Autodesk Fusion 360 part; units mm, degrees
(part 2 of 3)
  spline S17 degree 5 poles (8.5092, -53.844) (8.509, -53.837) (8.5085, -53.8231) (8.5078, -53.8022) (8.5068, -53.7744) (8.5054, -53.7397) (8.5038, -53.7051) (8.5021, -53.6705) (8.5002, -53.6359) (8.4982, -53.6014) (8.496, -53.567) (8.4936, -53.5327) (8.4911, -53.4983) (8.4885, -53.4641) (8.4857, -53.4299) (8.4827, -53.3958) (8.4796, -53.3617) (8.4763, -53.3277) (8.4729, -53.2938) (8.4693, -53.2599) (8.4656, -53.2261) (8.4617, -53.1924) (8.4576, -53.1587) (8.4534, -53.1251) (8.449, -53.0916) (8.4444, -53.0581) (8.4397, -53.0248) (8.4348, -52.9914) (8.4298, -52.9582) (8.4245, -52.925) (8.4191, -52.892) (8.4136, -52.859) (8.4078, -52.826) (8.4019, -52.7932) (8.3958, -52.7604) (8.3896, -52.7278) (8.3832, -52.6952) (8.3765, -52.6627) (8.3697, -52.6302) (8.3628, -52.5979) (8.3556, -52.5657) (8.3483, -52.5335) (8.3407, -52.5015) (8.333, -52.4695) (8.3251, -52.4377) (8.3169, -52.4059) (8.3086, -52.3743) (8.3001, -52.3428) (8.2914, -52.3113) (8.2825, -52.28) (8.2734, -52.2488) (8.2641, -52.2177) (8.2545, -52.1867) (8.2447, -52.1559) (8.2346, -52.1252) (8.2244, -52.0946) (8.2139, -52.0641) (8.2032, -52.0338) (8.1924, -52.0035) (8.1812, -51.9735) (8.1698, -51.9436) (8.158, -51.9139) (8.1459, -51.8844) (8.1334, -51.8551) (8.1205, -51.826) (8.1075, -51.7971) (8.0943, -51.7683) (8.0808, -51.7396) (8.0672, -51.7111) (8.0531, -51.6829) (8.0382, -51.6551) (8.0255, -51.6334) (8.0154, -51.6175) (8.0083, -51.6071) (8.0048, -51.6019) knots -1 -1 -1 -1 -1 -1 -0.98571429 -0.97142857 -0.95714286 -0.94285714 -0.92857143 -0.91428571 -0.9 -0.88571429 -0.87142857 -0.85714286 -0.84285714 -0.82857143 -0.81428571 -0.8 -0.78571429 -0.77142857 -0.75714286 -0.74285714 -0.72857143 -0.71428571 -0.7 -0.68571429 -0.67142857 -0.65714286 -0.64285714 -0.62857143 -0.61428571 -0.6 -0.58571429 -0.57142857 -0.55714286 -0.54285714 -0.52857143 -0.51428571 -0.5 -0.48571429 -0.47142857 -0.45714286 -0.44285714 -0.42857143 -0.41428571 -0.4 -0.38571429 -0.37142857 -0.35714286 -0.34285714 -0.32857143 -0.31428571 -0.3 -0.28571429 -0.27142857 -0.25714286 -0.24285714 -0.22857143 -0.21428571 -0.2 -0.18571429 -0.17142857 -0.15714286 -0.14285714 -0.12857143 -0.11428571 -0.1 -0.08571429 -0.07142857 -0.05714286 -0.04285714 -0.02857143 -0.01428571 0 0 0 0 0 0
  line L17 (8.0048, -51.6019) -> (7.7787, -51.2734)
  arc A35 (7.8389, -50.9285) -> (7.7787, -51.2734) centre (7.9847, -51.1316) ccw
  arc A36 (7.8389, -50.9285) -> (8.5272, -50.4003) centre (0, -40) ccw
  arc A37 (8.876, -50.4314) -> (8.5272, -50.4003) centre (8.6858, -50.5937) ccw
  line L18 (8.876, -50.4314) -> (9.1348, -50.7348)
  spline S18 degree 5 poles (9.1348, -50.7348) (9.1388, -50.7396) (9.1471, -50.7491) (9.1599, -50.7629) (9.1775, -50.7809) (9.2005, -50.8024) (9.2241, -50.8234) (9.2481, -50.8439) (9.2724, -50.8643) (9.2968, -50.8845) (9.3213, -50.9046) (9.3461, -50.9245) (9.3711, -50.9442) (9.3965, -50.9636) (9.4221, -50.9826) (9.448, -51.0014) (9.4742, -51.02) (9.5006, -51.0383) (9.5271, -51.0565) (9.5539, -51.0744) (9.5807, -51.0923) (9.6078, -51.1099) (9.635, -51.1274) (9.6625, -51.1446) (9.6901, -51.1617) (9.7179, -51.1786) (9.7458, -51.1953) (9.7739, -51.2119) (9.8022, -51.2282) (9.8306, -51.2444) (9.8592, -51.2605) (9.8879, -51.2764) (9.9168, -51.2921) (9.9458, -51.3077) (9.9749, -51.3231) (10.0042, -51.3384) (10.0336, -51.3535) (10.0632, -51.3685) (10.0929, -51.3833) (10.1227, -51.3979) (10.1526, -51.4124) (10.1827, -51.4268) (10.2129, -51.441) (10.2432, -51.455) (10.2736, -51.4689) (10.3042, -51.4827) (10.3349, -51.4963) (10.3657, -51.5098) (10.3966, -51.5232) (10.4276, -51.5364) (10.4588, -51.5494) (10.49, -51.5624) (10.5214, -51.5751) (10.5528, -51.5878) (10.5844, -51.6003) (10.6161, -51.6127) (10.6479, -51.6249) (10.6798, -51.637) (10.7118, -51.6489) (10.7438, -51.6608) (10.776, -51.6725) (10.8083, -51.684) (10.8407, -51.6954) (10.8732, -51.7067) (10.9058, -51.7179) (10.9385, -51.7289) (10.9713, -51.7398) (11.0042, -51.7505) (11.0371, -51.7612) (11.0702, -51.7717) (11.1033, -51.782) (11.1299, -51.7902) (11.1499, -51.7963) (11.1633, -51.8003) (11.1699, -51.8023) knots 0 0 0 0 0 0 0.01428571 0.02857143 0.04285714 0.05714286 0.07142857 0.08571429 0.1 0.11428571 0.12857143 0.14285714 0.15714286 0.17142857 0.18571429 0.2 0.21428571 0.22857143 0.24285714 0.25714286 0.27142857 0.28571429 0.3 0.31428571 0.32857143 0.34285714 0.35714286 0.37142857 0.38571429 0.4 0.41428571 0.42857143 0.44285714 0.45714286 0.47142857 0.48571429 0.5 0.51428571 0.52857143 0.54285714 0.55714286 0.57142857 0.58571429 0.6 0.61428571 0.62857143 0.64285714 0.65714286 0.67142857 0.68571429 0.7 0.71428571 0.72857143 0.74285714 0.75714286 0.77142857 0.78571429 0.8 0.81428571 0.82857143 0.84285714 0.85714286 0.87142857 0.88571429 0.9 0.91428571 0.92857143 0.94285714 0.95714286 0.97142857 0.98571429 1 1 1 1 1 1
  arc A38 (11.1699, -51.8023) -> (11.8023, -51.1699) centre (0, -40) ccw
  spline S19 degree 5 poles (11.8023, -51.1699) (11.8003, -51.1633) (11.7963, -51.1499) (11.7902, -51.1299) (11.782, -51.1033) (11.7717, -51.0702) (11.7612, -51.0371) (11.7505, -51.0042) (11.7398, -50.9713) (11.7289, -50.9385) (11.7179, -50.9058) (11.7067, -50.8732) (11.6954, -50.8407) (11.684, -50.8083) (11.6725, -50.776) (11.6608, -50.7438) (11.6489, -50.7118) (11.637, -50.6798) (11.6249, -50.6479) (11.6127, -50.6161) (11.6003, -50.5844) (11.5878, -50.5528) (11.5751, -50.5214) (11.5624, -50.49) (11.5494, -50.4588) (11.5364, -50.4276) (11.5232, -50.3966) (11.5098, -50.3657) (11.4963, -50.3349) (11.4827, -50.3042) (11.4689, -50.2736) (11.455, -50.2432) (11.441, -50.2129) (11.4268, -50.1827) (11.4124, -50.1526) (11.3979, -50.1227) (11.3833, -50.0929) (11.3685, -50.0632) (11.3535, -50.0336) (11.3384, -50.0042) (11.3231, -49.9749) (11.3077, -49.9458) (11.2921, -49.9168) (11.2764, -49.8879) (11.2605, -49.8592) (11.2444, -49.8306) (11.2282, -49.8022) (11.2119, -49.7739) (11.1953, -49.7458) (11.1786, -49.7179) (11.1617, -49.6901) (11.1446, -49.6625) (11.1274, -49.635) (11.1099, -49.6078) (11.0923, -49.5807) (11.0744, -49.5539) (11.0565, -49.5271) (11.0383, -49.5006) (11.02, -49.4742) (11.0014, -49.448) (10.9826, -49.4221) (10.9636, -49.3965) (10.9442, -49.3711) (10.9245, -49.3461) (10.9046, -49.3213) (10.8845, -49.2968) (10.8643, -49.2724) (10.8439, -49.2481) (10.8234, -49.2241) (10.8024, -49.2005) (10.7809, -49.1775) (10.7629, -49.1599) (10.7491, -49.1471) (10.7396, -49.1388) (10.7348, -49.1348) knots -1 -1 -1 -1 -1 -1 -0.98571429 -0.97142857 -0.95714286 -0.94285714 -0.92857143 -0.91428571 -0.9 -0.88571429 -0.87142857 -0.85714286 -0.84285714 -0.82857143 -0.81428571 -0.8 -0.78571429 -0.77142857 -0.75714286 -0.74285714 -0.72857143 -0.71428571 -0.7 -0.68571429 -0.67142857 -0.65714286 -0.64285714 -0.62857143 -0.61428571 -0.6 -0.58571429 -0.57142857 -0.55714286 -0.54285714 -0.52857143 -0.51428571 -0.5 -0.48571429 -0.47142857 -0.45714286 -0.44285714 -0.42857143 -0.41428571 -0.4 -0.38571429 -0.37142857 -0.35714286 -0.34285714 -0.32857143 -0.31428571 -0.3 -0.28571429 -0.27142857 -0.25714286 -0.24285714 -0.22857143 -0.21428571 -0.2 -0.18571429 -0.17142857 -0.15714286 -0.14285714 -0.12857143 -0.11428571 -0.1 -0.08571429 -0.07142857 -0.05714286 -0.04285714 -0.02857143 -0.01428571 0 0 0 0 0 0
  line L19 (10.7348, -49.1348) -> (10.4314, -48.876)
  arc A39 (10.4003, -48.5272) -> (10.4314, -48.876) centre (10.5937, -48.6858) ccw
  arc A40 (10.4003, -48.5272) -> (10.9285, -47.8389) centre (0, -40) ccw
  arc A41 (11.2734, -47.7787) -> (10.9285, -47.8389) centre (11.1316, -47.9847) ccw
  line L20 (11.2734, -47.7787) -> (11.6019, -48.0048)
  spline S20 degree 5 poles (11.6019, -48.0048) (11.6071, -48.0083) (11.6175, -48.0154) (11.6334, -48.0255) (11.6551, -48.0382) (11.6829, -48.0531) (11.7111, -48.0672) (11.7396, -48.0808) (11.7683, -48.0943) (11.7971, -48.1075) (11.826, -48.1205) (11.8551, -48.1334) (11.8844, -48.1459) (11.9139, -48.158) (11.9436, -48.1698) (11.9735, -48.1812) (12.0035, -48.1924) (12.0338, -48.2032) (12.0641, -48.2139) (12.0946, -48.2244) (12.1252, -48.2346) (12.1559, -48.2447) (12.1867, -48.2545) (12.2177, -48.2641) (12.2488, -48.2734) (12.28, -48.2825) (12.3113, -48.2914) (12.3428, -48.3001) (12.3743, -48.3086) (12.4059, -48.3169) (12.4377, -48.3251) (12.4695, -48.333) (12.5015, -48.3407) (12.5335, -48.3483) (12.5657, -48.3556) (12.5979, -48.3628) (12.6302, -48.3697) (12.6627, -48.3765) (12.6952, -48.3832) (12.7278, -48.3896) (12.7604, -48.3958) (12.7932, -48.4019) (12.826, -48.4078) (12.859, -48.4136) (12.892, -48.4191) (12.925, -48.4245) (12.9582, -48.4298) (12.9914, -48.4348) (13.0248, -48.4397) (13.0581, -48.4444) (13.0916, -48.449) (13.1251, -48.4534) (13.1587, -48.4576) (13.1924, -48.4617) (13.2261, -48.4656) (13.2599, -48.4693) (13.2938, -48.4729) (13.3277, -48.4763) (13.3617, -48.4796) (13.3958, -48.4827) (13.4299, -48.4857) (13.4641, -48.4885) (13.4983, -48.4911) (13.5327, -48.4936) (13.567, -48.496) (13.6014, -48.4982) (13.6359, -48.5002) (13.6705, -48.5021) (13.7051, -48.5038) (13.7397, -48.5054) (13.7744, -48.5068) (13.8022, -48.5078) (13.8231, -48.5085) (13.837, -48.509) (13.844, -48.5092) knots 0 0 0 0 0 0 0.01428571 0.02857143 0.04285714 0.05714286 0.07142857 0.08571429 0.1 0.11428571 0.12857143 0.14285714 0.15714286 0.17142857 0.18571429 0.2 0.21428571 0.22857143 0.24285714 0.25714286 0.27142857 0.28571429 0.3 0.31428571 0.32857143 0.34285714 0.35714286 0.37142857 0.38571429 0.4 0.41428571 0.42857143 0.44285714 0.45714286 0.47142857 0.48571429 0.5 0.51428571 0.52857143 0.54285714 0.55714286 0.57142857 0.58571429 0.6 0.61428571 0.62857143 0.64285714 0.65714286 0.67142857 0.68571429 0.7 0.71428571 0.72857143 0.74285714 0.75714286 0.77142857 0.78571429 0.8 0.81428571 0.82857143 0.84285714 0.85714286 0.87142857 0.88571429 0.9 0.91428571 0.92857143 0.94285714 0.95714286 0.97142857 0.98571429 1 1 1 1 1 1
  arc A42 (13.844, -48.5092) -> (14.2912, -47.7347) centre (0, -40) ccw
  spline S21 degree 5 poles (14.2912, -47.7347) (14.2875, -47.7287) (14.2802, -47.7169) (14.2691, -47.6992) (14.2543, -47.6756) (14.2357, -47.6463) (14.217, -47.617) (14.1982, -47.5879) (14.1793, -47.559) (14.1603, -47.5301) (14.1412, -47.5014) (14.122, -47.4728) (14.1027, -47.4443) (14.0833, -47.416) (14.0638, -47.3878) (14.0442, -47.3597) (14.0244, -47.3318) (14.0046, -47.304) (13.9847, -47.2763) (13.9646, -47.2488) (13.9445, -47.2214) (13.9242, -47.1941) (13.9039, -47.167) (13.8834, -47.14) (13.8628, -47.1132) (13.8422, -47.0865) (13.8214, -47.0599) (13.8005, -47.0335) (13.7795, -47.0073) (13.7584, -46.9812) (13.7372, -46.9552) (13.7158, -46.9294) (13.6944, -46.9038) (13.6729, -46.8783) (13.6512, -46.8529) (13.6295, -46.8278) (13.6076, -46.8028) (13.5856, -46.7779) (13.5635, -46.7532) (13.5413, -46.7287) (13.519, -46.7044) (13.4966, -46.6802) (13.474, -46.6562) (13.4514, -46.6324) (13.4286, -46.6088) (13.4057, -46.5854) (13.3826, -46.5621) (13.3595, -46.5391) (13.3362, -46.5162) (13.3129, -46.4935) (13.2894, -46.471) (13.2657, -46.4488) (13.2419, -46.4268) (13.218, -46.405) (13.194, -46.3834) (13.1698, -46.362) (13.1455, -46.3409) (13.1211, -46.3199) (13.0966, -46.2992) (13.0719, -46.2787) (13.047, -46.2585) (13.022, -46.2387) (12.9967, -46.2193) (12.9713, -46.2002) (12.9456, -46.1814) (12.9198, -46.1629) (12.894, -46.1445) (12.868, -46.1264) (12.8419, -46.1085) (12.8156, -46.0911) (12.7888, -46.0745) (12.767, -46.0621) (12.7503, -46.0534) (12.739, -46.0478) (12.7333, -46.0451) knots -1 -1 -1 -1 -1 -1 -0.98571429 -0.97142857 -0.95714286 -0.94285714 -0.92857143 -0.91428571 -0.9 -0.88571429 -0.87142857 -0.85714286 -0.84285714 -0.82857143 -0.81428571 -0.8 -0.78571429 -0.77142857 -0.75714286 -0.74285714 -0.72857143 -0.71428571 -0.7 -0.68571429 -0.67142857 -0.65714286 -0.64285714 -0.62857143 -0.61428571 -0.6 -0.58571429 -0.57142857 -0.55714286 -0.54285714 -0.52857143 -0.51428571 -0.5 -0.48571429 -0.47142857 -0.45714286 -0.44285714 -0.42857143 -0.41428571 -0.4 -0.38571429 -0.37142857 -0.35714286 -0.34285714 -0.32857143 -0.31428571 -0.3 -0.28571429 -0.27142857 -0.25714286 -0.24285714 -0.22857143 -0.21428571 -0.2 -0.18571429 -0.17142857 -0.15714286 -0.14285714 -0.12857143 -0.11428571 -0.1 -0.08571429 -0.07142857 -0.05714286 -0.04285714 -0.02857143 -0.01428571 0 0 0 0 0 0
  line L21 (12.7333, -46.0451) -> (12.3732, -45.8737)
  arc A43 (12.253, -45.5449) -> (12.3732, -45.8737) centre (12.4807, -45.648) ccw
  arc A44 (12.253, -45.5449) -> (12.585, -44.7433) centre (0, -40) ccw
  arc A45 (12.9025, -44.5959) -> (12.585, -44.7433) centre (12.8189, -44.8315) ccw
  line L22 (12.9025, -44.5959) -> (13.2783, -44.7292)
  spline S22 degree 5 poles (13.2783, -44.7292) (13.2843, -44.7313) (13.2962, -44.7354) (13.3142, -44.741) (13.3384, -44.7477) (13.3691, -44.7549) (13.4, -44.7613) (13.4311, -44.7671) (13.4623, -44.7726) (13.4935, -44.7779) (13.5248, -44.783) (13.5562, -44.7879) (13.5877, -44.7924) (13.6194, -44.7965) (13.6511, -44.8002) (13.6829, -44.8035) (13.7149, -44.8065) (13.7469, -44.8092) (13.779, -44.8116) (13.8111, -44.8138) (13.8433, -44.8158) (13.8756, -44.8176) (13.9079, -44.8191) (13.9403, -44.8203) (13.9727, -44.8213) (14.0052, -44.822) (14.0378, -44.8225) (14.0704, -44.8228) (14.1031, -44.8228) (14.1358, -44.8227) (14.1686, -44.8223) (14.2014, -44.8217) (14.2342, -44.8209) (14.2672, -44.8199) (14.3001, -44.8187) (14.3331, -44.8172) (14.3661, -44.8156) (14.3992, -44.8138) (14.4323, -44.8118) (14.4655, -44.8095) (14.4986, -44.8071) (14.5319, -44.8045) (14.5651, -44.8017) (14.5984, -44.7987) (14.6317, -44.7956) (14.6651, -44.7922) (14.6984, -44.7887) (14.7319, -44.785) (14.7653, -44.7811) (14.7988, -44.777) (14.8323, -44.7727) (14.8658, -44.7683) (14.8993, -44.7637) (14.9329, -44.7589) (14.9665, -44.754) (15.0001, -44.7488) (15.0338, -44.7435) (15.0674, -44.738) (15.1011, -44.7324) (15.1348, -44.7266) (15.1686, -44.7206) (15.2023, -44.7145) (15.2361, -44.7082) (15.2699, -44.7017) (15.3037, -44.6951) (15.3375, -44.6883) (15.3713, -44.6813) (15.4052, -44.6742) (15.439, -44.6669) (15.4729, -44.6595) (15.5068, -44.6519) (15.5339, -44.6457) (15.5543, -44.6409) (15.5678, -44.6377) (15.5746, -44.6361) knots 0 0 0 0 0 0 0.01428571 0.02857143 0.04285714 0.05714286 0.07142857 0.08571429 0.1 0.11428571 0.12857143 0.14285714 0.15714286 0.17142857 0.18571429 0.2 0.21428571 0.22857143 0.24285714 0.25714286 0.27142857 0.28571429 0.3 0.31428571 0.32857143 0.34285714 0.35714286 0.37142857 0.38571429 0.4 0.41428571 0.42857143 0.44285714 0.45714286 0.47142857 0.48571429 0.5 0.51428571 0.52857143 0.54285714 0.55714286 0.57142857 0.58571429 0.6 0.61428571 0.62857143 0.64285714 0.65714286 0.67142857 0.68571429 0.7 0.71428571 0.72857143 0.74285714 0.75714286 0.77142857 0.78571429 0.8 0.81428571 0.82857143 0.84285714 0.85714286 0.87142857 0.88571429 0.9 0.91428571 0.92857143 0.94285714 0.95714286 0.97142857 0.98571429 1 1 1 1 1 1
  arc A46 (15.5746, -44.6361) -> (15.8061, -43.7723) centre (0, -40) ccw
  spline S23 degree 5 poles (15.8061, -43.7723) (15.801, -43.7675) (15.7908, -43.758) (15.7756, -43.7437) (15.7552, -43.7248) (15.7297, -43.7012) (15.704, -43.6779) (15.6784, -43.6546) (15.6526, -43.6315) (15.6268, -43.6086) (15.6009, -43.5858) (15.5749, -43.5631) (15.5489, -43.5406) (15.5228, -43.5183) (15.4967, -43.4961) (15.4704, -43.4741) (15.4442, -43.4522) (15.4178, -43.4304) (15.3914, -43.4089) (15.3649, -43.3875) (15.3383, -43.3662) (15.3117, -43.3451) (15.285, -43.3242) (15.2583, -43.3034) (15.2315, -43.2828) (15.2046, -43.2624) (15.1777, -43.2421) (15.1506, -43.222) (15.1236, -43.2021) (15.0964, -43.1823) (15.0692, -43.1628) (15.042, -43.1434) (15.0146, -43.1241) (14.9872, -43.1051) (14.9597, -43.0862) (14.9322, -43.0675) (14.9046, -43.0491) (14.877, -43.0307) (14.8492, -43.0126) (14.8214, -42.9947) (14.7936, -42.977) (14.7657, -42.9594) (14.7377, -42.9421) (14.7096, -42.925) (14.6815, -42.9081) (14.6533, -42.8914) (14.625, -42.8749) (14.5967, -42.8586) (14.5683, -42.8425) (14.5399, -42.8266) (14.5114, -42.811) (14.4828, -42.7956) (14.4541, -42.7805) (14.4254, -42.7656) (14.3966, -42.751) (14.3677, -42.7367) (14.3387, -42.7225) (14.3097, -42.7086) (14.2807, -42.6949) (14.2515, -42.6815) (14.2223, -42.6685) (14.193, -42.6558) (14.1635, -42.6435) (14.134, -42.6317) (14.1044, -42.6202) (14.0747, -42.609) (14.0449, -42.5979) (14.0152, -42.5871) (13.9854, -42.5766) (13.9554, -42.5667) (13.9253, -42.5576) (13.9009, -42.5512) (13.8825, -42.5471) (13.8702, -42.5447) (13.864, -42.5435) knots -1 -1 -1 -1 -1 -1 -0.98571429 -0.97142857 -0.95714286 -0.94285714 -0.92857143 -0.91428571 -0.9 -0.88571429 -0.87142857 -0.85714286 -0.84285714 -0.82857143 -0.81428571 -0.8 -0.78571429 -0.77142857 -0.75714286 -0.74285714 -0.72857143 -0.71428571 -0.7 -0.68571429 -0.67142857 -0.65714286 -0.64285714 -0.62857143 -0.61428571 -0.6 -0.58571429 -0.57142857 -0.55714286 -0.54285714 -0.52857143 -0.51428571 -0.5 -0.48571429 -0.47142857 -0.45714286 -0.44285714 -0.42857143 -0.41428571 -0.4 -0.38571429 -0.37142857 -0.35714286 -0.34285714 -0.32857143 -0.31428571 -0.3 -0.28571429 -0.27142857 -0.25714286 -0.24285714 -0.22857143 -0.21428571 -0.2 -0.18571429 -0.17142857 -0.15714286 -0.14285714 -0.12857143 -0.11428571 -0.1 -0.08571429 -0.07142857 -0.05714286 -0.04285714 -0.02857143 -0.01428571 0 0 0 0 0 0
  line L23 (13.864, -42.5435) -> (13.4718, -42.4711)
  arc A47 (13.2706, -42.1846) -> (13.4718, -42.4711) centre (13.5173, -42.2252) ccw
  arc A48 (13.2706, -42.1846) -> (13.3838, -41.3245) centre (0, -40) ccw
  arc A49 (13.6524, -41.0999) -> (13.3838, -41.3245) centre (13.6326, -41.3491) ccw
  line L24 (13.6524, -41.0999) -> (14.0499, -41.1314)
  spline S24 degree 5 poles (14.0499, -41.1314) (14.0562, -41.1319) (14.0687, -41.1327) (14.0876, -41.1335) (14.1127, -41.1337) (14.1442, -41.1327) (14.1757, -41.1308) (14.2072, -41.1284) (14.2388, -41.1257) (14.2703, -41.1227) (14.3019, -41.1196) (14.3335, -41.1161) (14.3651, -41.1123) (14.3967, -41.1081) (14.4283, -41.1035) (14.4599, -41.0984) (14.4916, -41.093) (14.5232, -41.0873) (14.5548, -41.0814) (14.5864, -41.0752) (14.618, -41.0688) (14.6496, -41.0622) (14.6812, -41.0552) (14.7128, -41.048) (14.7444, -41.0406) (14.776, -41.0329) (14.8076, -41.0249) (14.8392, -41.0168) (14.8708, -41.0083) (14.9023, -40.9997) (14.9339, -40.9909) (14.9654, -40.9818) (14.997, -40.9725) (15.0285, -40.963) (15.06, -40.9533) (15.0915, -40.9434) (15.123, -40.9333) (15.1545, -40.923) (15.1859, -40.9124) (15.2174, -40.9017) (15.2488, -40.8908) (15.2802, -40.8797) (15.3116, -40.8684) (15.343, -40.8569) (15.3743, -40.8452) (15.4057, -40.8333) (15.437, -40.8213) (15.4683, -40.809) (15.4996, -40.7966) (15.5309, -40.784) (15.5621, -40.7712) (15.5934, -40.7583) (15.6246, -40.7451) (15.6558, -40.7318) (15.6869, -40.7183) (15.7181, -40.7047) (15.7492, -40.6909) (15.7803, -40.6769) (15.8114, -40.6627) (15.8425, -40.6484) (15.8735, -40.6339) (15.9045, -40.6192) (15.9355, -40.6044) (15.9664, -40.5894) (15.9974, -40.5742) (16.0283, -40.5589) (16.0592, -40.5434) (16.09, -40.5278) (16.1208, -40.512) (16.1516, -40.496) (16.1824, -40.4799) (16.207, -40.4669) (16.2254, -40.4571) (16.2377, -40.4505) (16.2438, -40.4472) knots 0 0 0 0 0 0 0.01428571 0.02857143 0.04285714 0.05714286 0.07142857 0.08571429 0.1 0.11428571 0.12857143 0.14285714 0.15714286 0.17142857 0.18571429 0.2 0.21428571 0.22857143 0.24285714 0.25714286 0.27142857 0.28571429 0.3 0.31428571 0.32857143 0.34285714 0.35714286 0.37142857 0.38571429 0.4 0.41428571 0.42857143 0.44285714 0.45714286 0.47142857 0.48571429 0.5 0.51428571 0.52857143 0.54285714 0.55714286 0.57142857 0.58571429 0.6 0.61428571 0.62857143 0.64285714 0.65714286 0.67142857 0.68571429 0.7 0.71428571 0.72857143 0.74285714 0.75714286 0.77142857 0.78571429 0.8 0.81428571 0.82857143 0.84285714 0.85714286 0.87142857 0.88571429 0.9 0.91428571 0.92857143 0.94285714 0.95714286 0.97142857 0.98571429 1 1 1 1 1 1
  arc A50 (16.2438, -40.4472) -> (16.2438, -39.5528) centre (0, -40) ccw
  spline S25 degree 5 poles (16.2438, -39.5528) (16.2377, -39.5495) (16.2254, -39.5429) (16.207, -39.5331) (16.1824, -39.5201) (16.1516, -39.504) (16.1208, -39.488) (16.09, -39.4722) (16.0592, -39.4566) (16.0283, -39.4411) (15.9974, -39.4258) (15.9664, -39.4106) (15.9355, -39.3956) (15.9045, -39.3808) (15.8735, -39.3661) (15.8425, -39.3516) (15.8114, -39.3373) (15.7803, -39.3231) (15.7492, -39.3091) (15.7181, -39.2953) (15.6869, -39.2817) (15.6558, -39.2682) (15.6246, -39.2549) (15.5934, -39.2417) (15.5621, -39.2288) (15.5309, -39.216) (15.4996, -39.2034) (15.4683, -39.191) (15.437, -39.1787) (15.4057, -39.1667) (15.3743, -39.1548) (15.343, -39.1431) (15.3116, -39.1316) (15.2802, -39.1203) (15.2488, -39.1092) (15.2174, -39.0983) (15.1859, -39.0876) (15.1545, -39.077) (15.123, -39.0667) (15.0915, -39.0566) (15.06, -39.0467) (15.0285, -39.037) (14.997, -39.0275) (14.9654, -39.0182) (14.9339, -39.0091) (14.9023, -39.0003) (14.8708, -38.9917) (14.8392, -38.9832) (14.8076, -38.9751) (14.776, -38.9671) (14.7444, -38.9594) (14.7128, -38.952) (14.6812, -38.9448) (14.6496, -38.9378) (14.618, -38.9312) (14.5864, -38.9248) (14.5548, -38.9186) (14.5232, -38.9127) (14.4916, -38.907) (14.4599, -38.9016) (14.4283, -38.8965) (14.3967, -38.8919) (14.3651, -38.8877) (14.3335, -38.8839) (14.3019, -38.8804) (14.2703, -38.8773) (14.2388, -38.8743) (14.2072, -38.8716) (14.1757, -38.8692) (14.1442, -38.8673) (14.1127, -38.8663) (14.0876, -38.8665) (14.0687, -38.8673) (14.0562, -38.8681) (14.0499, -38.8686) knots -1 -1 -1 -1 -1 -1 -0.98571429 -0.97142857 -0.95714286 -0.94285714 -0.92857143 -0.91428571 -0.9 -0.88571429 -0.87142857 -0.85714286 -0.84285714 -0.82857143 -0.81428571 -0.8 -0.78571429 -0.77142857 -0.75714286 -0.74285714 -0.72857143 -0.71428571 -0.7 -0.68571429 -0.67142857 -0.65714286 -0.64285714 -0.62857143 -0.61428571 -0.6 -0.58571429 -0.57142857 -0.55714286 -0.54285714 -0.52857143 -0.51428571 -0.5 -0.48571429 -0.47142857 -0.45714286 -0.44285714 -0.42857143 -0.41428571 -0.4 -0.38571429 -0.37142857 -0.35714286 -0.34285714 -0.32857143 -0.31428571 -0.3 -0.28571429 -0.27142857 -0.25714286 -0.24285714 -0.22857143 -0.21428571 -0.2 -0.18571429 -0.17142857 -0.15714286 -0.14285714 -0.12857143 -0.11428571 -0.1 -0.08571429 -0.07142857 -0.05714286 -0.04285714 -0.02857143 -0.01428571 0 0 0 0 0 0
  line L25 (14.0499, -38.8686) -> (13.6524, -38.9001)
  arc A51 (13.3838, -38.6755) -> (13.6524, -38.9001) centre (13.6326, -38.6509) ccw
  arc A52 (13.3838, -38.6755) -> (13.2706, -37.8154) centre (0, -40) ccw
  arc A53 (13.4718, -37.5289) -> (13.2706, -37.8154) centre (13.5173, -37.7748) ccw
  line L26 (13.4718, -37.5289) -> (13.864, -37.4565)
  spline S26 degree 5 poles (13.864, -37.4565) (13.8702, -37.4553) (13.8825, -37.4529) (13.9009, -37.4488) (13.9253, -37.4424) (13.9554, -37.4333) (13.9854, -37.4234) (14.0152, -37.4129) (14.0449, -37.4021) (14.0747, -37.391) (14.1044, -37.3798) (14.134, -37.3683) (14.1635, -37.3565) (14.193, -37.3442) (14.2223, -37.3315) (14.2515, -37.3185) (14.2807, -37.3051) (14.3097, -37.2914) (14.3387, -37.2775) (14.3677, -37.2633) (14.3966, -37.249) (14.4254, -37.2344) (14.4541, -37.2195) (14.4828, -37.2044) (14.5114, -37.189) (14.5399, -37.1734) (14.5683, -37.1575) (14.5967, -37.1414) (14.625, -37.1251) (14.6533, -37.1086) (14.6815, -37.0919) (14.7096, -37.075) (14.7377, -37.0579) (14.7657, -37.0406) (14.7936, -37.023) (14.8214, -37.0053) (14.8492, -36.9874) (14.877, -36.9693) (14.9046, -36.9509) (14.9322, -36.9325) (14.9597, -36.9138) (14.9872, -36.8949) (15.0146, -36.8759) (15.042, -36.8566) (15.0692, -36.8372) (15.0964, -36.8177) (15.1236, -36.7979) (15.1506, -36.778) (15.1777, -36.7579) (15.2046, -36.7376) (15.2315, -36.7172) (15.2583, -36.6966) (15.285, -36.6758) (15.3117, -36.6549) (15.3383, -36.6338) (15.3649, -36.6125) (15.3914, -36.5911) (15.4178, -36.5696) (15.4442, -36.5478) (15.4704, -36.5259) (15.4967, -36.5039) (15.5228, -36.4817) (15.5489, -36.4594) (15.5749, -36.4369) (15.6009, -36.4142) (15.6268, -36.3914) (15.6526, -36.3685) (15.6784, -36.3454) (15.704, -36.3221) (15.7297, -36.2988) (15.7552, -36.2752) (15.7756, -36.2563) (15.7908, -36.242) (15.801, -36.2325) (15.8061, -36.2277) knots 0 0 0 0 0 0 0.01428571 0.02857143 0.04285714 0.05714286 0.07142857 0.08571429 0.1 0.11428571 0.12857143 0.14285714 0.15714286 0.17142857 0.18571429 0.2 0.21428571 0.22857143 0.24285714 0.25714286 0.27142857 0.28571429 0.3 0.31428571 0.32857143 0.34285714 0.35714286 0.37142857 0.38571429 0.4 0.41428571 0.42857143 0.44285714 0.45714286 0.47142857 0.48571429 0.5 0.51428571 0.52857143 0.54285714 0.55714286 0.57142857 0.58571429 0.6 0.61428571 0.62857143 0.64285714 0.65714286 0.67142857 0.68571429 0.7 0.71428571 0.72857143 0.74285714 0.75714286 0.77142857 0.78571429 0.8 0.81428571 0.82857143 0.84285714 0.85714286 0.87142857 0.88571429 0.9 0.91428571 0.92857143 0.94285714 0.95714286 0.97142857 0.98571429 1 1 1 1 1 1
  arc A54 (15.8061, -36.2277) -> (15.5746, -35.3639) centre (0, -40) ccw
  spline S27 degree 5 poles (15.5746, -35.3639) (15.5678, -35.3623) (15.5543, -35.3591) (15.5339, -35.3543) (15.5068, -35.3481) (15.4729, -35.3405) (15.439, -35.3331) (15.4052, -35.3258) (15.3713, -35.3187) (15.3375, -35.3117) (15.3037, -35.3049) (15.2699, -35.2983) (15.2361, -35.2918) (15.2023, -35.2855) (15.1686, -35.2794) (15.1348, -35.2734) (15.1011, -35.2676) (15.0674, -35.262) (15.0338, -35.2565) (15.0001, -35.2512) (14.9665, -35.246) (14.9329, -35.2411) (14.8993, -35.2363) (14.8658, -35.2317) (14.8323, -35.2273) (14.7988, -35.223) (14.7653, -35.2189) (14.7319, -35.215) (14.6984, -35.2113) (14.6651, -35.2078) (14.6317, -35.2044) (14.5984, -35.2013) (14.5651, -35.1983) (14.5319, -35.1955) (14.4986, -35.1929) (14.4655, -35.1905) (14.4323, -35.1882) (14.3992, -35.1862) (14.3661, -35.1844) (14.3331, -35.1828) (14.3001, -35.1813) (14.2672, -35.1801) (14.2342, -35.1791) (14.2014, -35.1783) (14.1686, -35.1777) (14.1358, -35.1773) (14.1031, -35.1772) (14.0704, -35.1772) (14.0378, -35.1775) (14.0052, -35.178) (13.9727, -35.1787) (13.9403, -35.1797) (13.9079, -35.1809) (13.8756, -35.1824) (13.8433, -35.1842) (13.8111, -35.1862) (13.779, -35.1884) (13.7469, -35.1908) (13.7149, -35.1935) (13.6829, -35.1965) (13.6511, -35.1998) (13.6194, -35.2035) (13.5877, -35.2076) (13.5562, -35.2121) (13.5248, -35.217) (13.4935, -35.2221) (13.4623, -35.2274) (13.4311, -35.2329) (13.4, -35.2387) (13.3691, -35.2451) (13.3384, -35.2523) (13.3142, -35.259) (13.2962, -35.2646) (13.2843, -35.2687) (13.2783, -35.2708) knots -1 -1 -1 -1 -1 -1 -0.98571429 -0.97142857 -0.95714286 -0.94285714 -0.92857143 -0.91428571 -0.9 -0.88571429 -0.87142857 -0.85714286 -0.84285714 -0.82857143 -0.81428571 -0.8 -0.78571429 -0.77142857 -0.75714286 -0.74285714 -0.72857143 -0.71428571 -0.7 -0.68571429 -0.67142857 -0.65714286 -0.64285714 -0.62857143 -0.61428571 -0.6 -0.58571429 -0.57142857 -0.55714286 -0.54285714 -0.52857143 -0.51428571 -0.5 -0.48571429 -0.47142857 -0.45714286 -0.44285714 -0.42857143 -0.41428571 -0.4 -0.38571429 -0.37142857 -0.35714286 -0.34285714 -0.32857143 -0.31428571 -0.3 -0.28571429 -0.27142857 -0.25714286 -0.24285714 -0.22857143 -0.21428571 -0.2 -0.18571429 -0.17142857 -0.15714286 -0.14285714 -0.12857143 -0.11428571 -0.1 -0.08571429 -0.07142857 -0.05714286 -0.04285714 -0.02857143 -0.01428571 0 0 0 0 0 0
  line L27 (13.2783, -35.2708) -> (12.9025, -35.4041)
  arc A55 (12.585, -35.2567) -> (12.9025, -35.4041) centre (12.8189, -35.1685) ccw
  arc A56 (12.585, -35.2567) -> (12.253, -34.4551) centre (0, -40) ccw
  arc A57 (12.3732, -34.1263) -> (12.253, -34.4551) centre (12.4807, -34.352) ccw
  line L28 (12.3732, -34.1263) -> (12.7333, -33.9549)
  spline S28 degree 5 poles (12.7333, -33.9549) (12.739, -33.9522) (12.7503, -33.9466) (12.767, -33.9379) (12.7888, -33.9255) (12.8156, -33.9089) (12.8419, -33.8915) (12.868, -33.8736) (12.894, -33.8555) (12.9198, -33.8371) (12.9456, -33.8186) (12.9713, -33.7998) (12.9967, -33.7807) (13.022, -33.7613) (13.047, -33.7415) (13.0719, -33.7213) (13.0966, -33.7008) (13.1211, -33.6801) (13.1455, -33.6591) (13.1698, -33.638) (13.194, -33.6166) (13.218, -33.595) (13.2419, -33.5732) (13.2657, -33.5512) (13.2894, -33.529) (13.3129, -33.5065) (13.3362, -33.4838) (13.3595, -33.4609) (13.3826, -33.4379) (13.4057, -33.4146) (13.4286, -33.3912) (13.4514, -33.3676) (13.474, -33.3438) (13.4966, -33.3198) (13.519, -33.2956) (13.5413, -33.2713) (13.5635, -33.2468) (13.5856, -33.2221) (13.6076, -33.1972) (13.6295, -33.1722) (13.6512, -33.1471) (13.6729, -33.1217) (13.6944, -33.0962) (13.7158, -33.0706) (13.7372, -33.0448) (13.7584, -33.0188) (13.7795, -32.9927) (13.8005, -32.9665) (13.8214, -32.9401) (13.8422, -32.9135) (13.8628, -32.8868) (13.8834, -32.86) (13.9039, -32.833) (13.9242, -32.8059) (13.9445, -32.7786) (13.9646, -32.7512) (13.9847, -32.7237) (14.0046, -32.696) (14.0244, -32.6682) (14.0442, -32.6403) (14.0638, -32.6122) (14.0833, -32.584) (14.1027, -32.5557) (14.122, -32.5272) (14.1412, -32.4986) (14.1603, -32.4699) (14.1793, -32.441) (14.1982, -32.4121) (14.217, -32.383) (14.2357, -32.3537) (14.2543, -32.3244) (14.2691, -32.3008) (14.2802, -32.2831) (14.2875, -32.2713) (14.2912, -32.2653) knots 0 0 0 0 0 0 0.01428571 0.02857143 0.04285714 0.05714286 0.07142857 0.08571429 0.1 0.11428571 0.12857143 0.14285714 0.15714286 0.17142857 0.18571429 0.2 0.21428571 0.22857143 0.24285714 0.25714286 0.27142857 0.28571429 0.3 0.31428571 0.32857143 0.34285714 0.35714286 0.37142857 0.38571429 0.4 0.41428571 0.42857143 0.44285714 0.45714286 0.47142857 0.48571429 0.5 0.51428571 0.52857143 0.54285714 0.55714286 0.57142857 0.58571429 0.6 0.61428571 0.62857143 0.64285714 0.65714286 0.67142857 0.68571429 0.7 0.71428571 0.72857143 0.74285714 0.75714286 0.77142857 0.78571429 0.8 0.81428571 0.82857143 0.84285714 0.85714286 0.87142857 0.88571429 0.9 0.91428571 0.92857143 0.94285714 0.95714286 0.97142857 0.98571429 1 1 1 1 1 1
  arc A58 (14.2912, -32.2653) -> (13.844, -31.4908) centre (0, -40) ccw
  spline S29 degree 5 poles (13.844, -31.4908) (13.837, -31.491) (13.8231, -31.4915) (13.8022, -31.4922) (13.7744, -31.4932) (13.7397, -31.4946) (13.7051, -31.4962) (13.6705, -31.4979) (13.6359, -31.4998) (13.6014, -31.5018) (13.567, -31.504) (13.5327, -31.5064) (13.4983, -31.5089) (13.4641, -31.5115) (13.4299, -31.5143) (13.3958, -31.5173) (13.3617, -31.5204) (13.3277, -31.5237) (13.2938, -31.5271) (13.2599, -31.5307) (13.2261, -31.5344) (13.1924, -31.5383) (13.1587, -31.5424) (13.1251, -31.5466) (13.0916, -31.551) (13.0581, -31.5556) (13.0248, -31.5603) (12.9914, -31.5652) (12.9582, -31.5702) (12.925, -31.5755) (12.892, -31.5809) (12.859, -31.5864) (12.826, -31.5922) (12.7932, -31.5981) (12.7604, -31.6042) (12.7278, -31.6104) (12.6952, -31.6168) (12.6627, -31.6235) (12.6302, -31.6303) (12.5979, -31.6372) (12.5657, -31.6444) (12.5335, -31.6517) (12.5015, -31.6593) (12.4695, -31.667) (12.4377, -31.6749) (12.4059, -31.6831) (12.3743, -31.6914) (12.3428, -31.6999) (12.3113, -31.7086) (12.28, -31.7175) (12.2488, -31.7266) (12.2177, -31.7359) (12.1867, -31.7455) (12.1559, -31.7553) (12.1252, -31.7654) (12.0946, -31.7756) (12.0641, -31.7861) (12.0338, -31.7968) (12.0035, -31.8076) (11.9735, -31.8188) (11.9436, -31.8302) (11.9139, -31.842) (11.8844, -31.8541) (11.8551, -31.8666) (11.826, -31.8795) (11.7971, -31.8925) (11.7683, -31.9057) (11.7396, -31.9192) (11.7111, -31.9328) (11.6829, -31.9469) (11.6551, -31.9618) (11.6334, -31.9745) (11.6175, -31.9846) (11.6071, -31.9917) (11.6019, -31.9952) knots -1 -1 -1 -1 -1 -1 -0.98571429 -0.97142857 -0.95714286 -0.94285714 -0.92857143 -0.91428571 -0.9 -0.88571429 -0.87142857 -0.85714286 -0.84285714 -0.82857143 -0.81428571 -0.8 -0.78571429 -0.77142857 -0.75714286 -0.74285714 -0.72857143 -0.71428571 -0.7 -0.68571429 -0.67142857 -0.65714286 -0.64285714 -0.62857143 -0.61428571 -0.6 -0.58571429 -0.57142857 -0.55714286 -0.54285714 -0.52857143 -0.51428571 -0.5 -0.48571429 -0.47142857 -0.45714286 -0.44285714 -0.42857143 -0.41428571 -0.4 -0.38571429 -0.37142857 -0.35714286 -0.34285714 -0.32857143 -0.31428571 -0.3 -0.28571429 -0.27142857 -0.25714286 -0.24285714 -0.22857143 -0.21428571 -0.2 -0.18571429 -0.17142857 -0.15714286 -0.14285714 -0.12857143 -0.11428571 -0.1 -0.08571429 -0.07142857 -0.05714286 -0.04285714 -0.02857143 -0.01428571 0 0 0 0 0 0
  line L29 (11.6019, -31.9952) -> (11.2734, -32.2213)
  arc A59 (10.9285, -32.1611) -> (11.2734, -32.2213) centre (11.1316, -32.0153) ccw
  arc A60 (10.9285, -32.1611) -> (10.4003, -31.4728) centre (0, -40) ccw
  arc A61 (10.4314, -31.124) -> (10.4003, -31.4728) centre (10.5937, -31.3142) ccw
  line L30 (10.4314, -31.124) -> (10.7348, -30.8652)
  spline S30 degree 5 poles (10.7348, -30.8652) (10.7396, -30.8612) (10.7491, -30.8529) (10.7629, -30.8401) (10.7809, -30.8225) (10.8024, -30.7995) (10.8234, -30.7759) (10.8439, -30.7519) (10.8643, -30.7276) (10.8845, -30.7032) (10.9046, -30.6787) (10.9245, -30.6539) (10.9442, -30.6289) (10.9636, -30.6035) (10.9826, -30.5779) (11.0014, -30.552) (11.02, -30.5258) (11.0383, -30.4994) (11.0565, -30.4729) (11.0744, -30.4461) (11.0923, -30.4193) (11.1099, -30.3922) (11.1274, -30.365) (11.1446, -30.3375) (11.1617, -30.3099) (11.1786, -30.2821) (11.1953, -30.2542) (11.2119, -30.2261) (11.2282, -30.1978) (11.2444, -30.1694) (11.2605, -30.1408) (11.2764, -30.1121) (11.2921, -30.0832) (11.3077, -30.0542) (11.3231, -30.0251) (11.3384, -29.9958) (11.3535, -29.9664) (11.3685, -29.9368) (11.3833, -29.9071) (11.3979, -29.8773) (11.4124, -29.8474) (11.4268, -29.8173) (11.441, -29.7871) (11.455, -29.7568) (11.4689, -29.7264) (11.4827, -29.6958) (11.4963, -29.6651) (11.5098, -29.6343) (11.5232, -29.6034) (11.5364, -29.5724) (11.5494, -29.5412) (11.5624, -29.51) (11.5751, -29.4786) (11.5878, -29.4472) (11.6003, -29.4156) (11.6127, -29.3839) (11.6249, -29.3521) (11.637, -29.3202) (11.6489, -29.2882) (11.6608, -29.2562) (11.6725, -29.224) (11.684, -29.1917) (11.6954, -29.1593) (11.7067, -29.1268) (11.7179, -29.0942) (11.7289, -29.0615) (11.7398, -29.0287) (11.7505, -28.9958) (11.7612, -28.9629) (11.7717, -28.9298) (11.782, -28.8967) (11.7902, -28.8701) (11.7963, -28.8501) (11.8003, -28.8367) (11.8023, -28.8301) knots 0 0 0 0 0 0 0.01428571 0.02857143 0.04285714 0.05714286 0.07142857 0.08571429 0.1 0.11428571 0.12857143 0.14285714 0.15714286 0.17142857 0.18571429 0.2 0.21428571 0.22857143 0.24285714 0.25714286 0.27142857 0.28571429 0.3 0.31428571 0.32857143 0.34285714 0.35714286 0.37142857 0.38571429 0.4 0.41428571 0.42857143 0.44285714 0.45714286 0.47142857 0.48571429 0.5 0.51428571 0.52857143 0.54285714 0.55714286 0.57142857 0.58571429 0.6 0.61428571 0.62857143 0.64285714 0.65714286 0.67142857 0.68571429 0.7 0.71428571 0.72857143 0.74285714 0.75714286 0.77142857 0.78571429 0.8 0.81428571 0.82857143 0.84285714 0.85714286 0.87142857 0.88571429 0.9 0.91428571 0.92857143 0.94285714 0.95714286 0.97142857 0.98571429 1 1 1 1 1 1
  arc A62 (11.8023, -28.8301) -> (11.1699, -28.1977) centre (0, -40) ccw
  spline S31 degree 5 poles (11.1699, -28.1977) (11.1633, -28.1997) (11.1499, -28.2037) (11.1299, -28.2098) (11.1033, -28.218) (11.0702, -28.2283) (11.0371, -28.2388) (11.0042, -28.2495) (10.9713, -28.2602) (10.9385, -28.2711) (10.9058, -28.2821) (10.8732, -28.2933) (10.8407, -28.3046) (10.8083, -28.316) (10.776, -28.3275) (10.7438, -28.3392) (10.7118, -28.3511) (10.6798, -28.363) (10.6479, -28.3751) (10.6161, -28.3873) (10.5844, -28.3997) (10.5528, -28.4122) (10.5214, -28.4249) (10.49, -28.4376) (10.4588, -28.4506) (10.4276, -28.4636) (10.3966, -28.4768) (10.3657, -28.4902) (10.3349, -28.5037) (10.3042, -28.5173) (10.2736, -28.5311) (10.2432, -28.545) (10.2129, -28.559) (10.1827, -28.5732) (10.1526, -28.5876) (10.1227, -28.6021) (10.0929, -28.6167) (10.0632, -28.6315) (10.0336, -28.6465) (10.0042, -28.6616) (9.9749, -28.6769) (9.9458, -28.6923) (9.9168, -28.7079) (9.8879, -28.7236) (9.8592, -28.7395) (9.8306, -28.7556) (9.8022, -28.7718) (9.7739, -28.7881) (9.7458, -28.8047) (9.7179, -28.8214) (9.6901, -28.8383) (9.6625, -28.8554) (9.635, -28.8726) (9.6078, -28.8901) (9.5807, -28.9077) (9.5539, -28.9256) (9.5271, -28.9435) (9.5006, -28.9617) (9.4742, -28.98) (9.448, -28.9986) (9.4221, -29.0174) (9.3965, -29.0364) (9.3711, -29.0558) (9.3461, -29.0755) (9.3213, -29.0954) (9.2968, -29.1155) (9.2724, -29.1357) (9.2481, -29.1561) (9.2241, -29.1766) (9.2005, -29.1976) (9.1775, -29.2191) (9.1599, -29.2371) (9.1471, -29.2509) (9.1388, -29.2604) (9.1348, -29.2652) knots -1 -1 -1 -1 -1 -1 -0.98571429 -0.97142857 -0.95714286 -0.94285714 -0.92857143 -0.91428571 -0.9 -0.88571429 -0.87142857 -0.85714286 -0.84285714 -0.82857143 -0.81428571 -0.8 -0.78571429 -0.77142857 -0.75714286 -0.74285714 -0.72857143 -0.71428571 -0.7 -0.68571429 -0.67142857 -0.65714286 -0.64285714 -0.62857143 -0.61428571 -0.6 -0.58571429 -0.57142857 -0.55714286 -0.54285714 -0.52857143 -0.51428571 -0.5 -0.48571429 -0.47142857 -0.45714286 -0.44285714 -0.42857143 -0.41428571 -0.4 -0.38571429 -0.37142857 -0.35714286 -0.34285714 -0.32857143 -0.31428571 -0.3 -0.28571429 -0.27142857 -0.25714286 -0.24285714 -0.22857143 -0.21428571 -0.2 -0.18571429 -0.17142857 -0.15714286 -0.14285714 -0.12857143 -0.11428571 -0.1 -0.08571429 -0.07142857 -0.05714286 -0.04285714 -0.02857143 -0.01428571 0 0 0 0 0 0
  line L31 (9.1348, -29.2652) -> (8.876, -29.5686)
  arc A63 (8.5272, -29.5997) -> (8.876, -29.5686) centre (8.6858, -29.4063) ccw
  arc A64 (8.5272, -29.5997) -> (7.8389, -29.0715) centre (0, -40) ccw
  arc A65 (7.7787, -28.7266) -> (7.8389, -29.0715) centre (7.9847, -28.8684) ccw
  line L32 (7.7787, -28.7266) -> (8.0048, -28.3981)
  spline S32 degree 5 poles (8.0048, -28.3981) (8.0083, -28.3929) (8.0154, -28.3825) (8.0255, -28.3666) (8.0382, -28.3449) (8.0531, -28.3171) (8.0672, -28.2889) (8.0808, -28.2604) (8.0943, -28.2317) (8.1075, -28.2029) (8.1205, -28.174) (8.1334, -28.1449) (8.1459, -28.1156) (8.158, -28.0861) (8.1698, -28.0564) (8.1812, -28.0265) (8.1924, -27.9965) (8.2032, -27.9662) (8.2139, -27.9359) (8.2244, -27.9054) (8.2346, -27.8748) (8.2447, -27.8441) (8.2545, -27.8133) (8.2641, -27.7823) (8.2734, -27.7512) (8.2825, -27.72) (8.2914, -27.6887) (8.3001, -27.6572) (8.3086, -27.6257) (8.3169, -27.5941) (8.3251, -27.5623) (8.333, -27.5305) (8.3407, -27.4985) (8.3483, -27.4665) (8.3556, -27.4343) (8.3628, -27.4021) (8.3697, -27.3698) (8.3765, -27.3373) (8.3832, -27.3048) (8.3896, -27.2722) (8.3958, -27.2396) (8.4019, -27.2068) (8.4078, -27.174) (8.4136, -27.141) (8.4191, -27.108) (8.4245, -27.075) (8.4298, -27.0418) (8.4348, -27.0086) (8.4397, -26.9752) (8.4444, -26.9419) (8.449, -26.9084) (8.4534, -26.8749) (8.4576, -26.8413) (8.4617, -26.8076) (8.4656, -26.7739) (8.4693, -26.7401) (8.4729, -26.7062) (8.4763, -26.6723) (8.4796, -26.6383) (8.4827, -26.6042) (8.4857, -26.5701) (8.4885, -26.5359) (8.4911, -26.5017) (8.4936, -26.4673) (8.496, -26.433) (8.4982, -26.3986) (8.5002, -26.3641) (8.5021, -26.3295) (8.5038, -26.2949) (8.5054, -26.2603) (8.5068, -26.2256) (8.5078, -26.1978) (8.5085, -26.1769) (8.509, -26.163) (8.5092, -26.156) knots 0 0 0 0 0 0 0.01428571 0.02857143 0.04285714 0.05714286 0.07142857 0.08571429 0.1 0.11428571 0.12857143 0.14285714 0.15714286 0.17142857 0.18571429 0.2 0.21428571 0.22857143 0.24285714 0.25714286 0.27142857 0.28571429 0.3 0.31428571 0.32857143 0.34285714 0.35714286 0.37142857 0.38571429 0.4 0.41428571 0.42857143 0.44285714 0.45714286 0.47142857 0.48571429 0.5 0.51428571 0.52857143 0.54285714 0.55714286 0.57142857 0.58571429 0.6 0.61428571 0.62857143 0.64285714 0.65714286 0.67142857 0.68571429 0.7 0.71428571 0.72857143 0.74285714 0.75714286 0.77142857 0.78571429 0.8 0.81428571 0.82857143 0.84285714 0.85714286 0.87142857 0.88571429 0.9 0.91428571 0.92857143 0.94285714 0.95714286 0.97142857 0.98571429 1 1 1 1 1 1
  arc A66 (8.5092, -26.156) -> (7.7347, -25.7088) centre (0, -40) ccw
  spline S33 degree 5 poles (7.7347, -25.7088) (7.7287, -25.7125) (7.7169, -25.7198) (7.6992, -25.7309) (7.6756, -25.7457) (7.6463, -25.7643) (7.617, -25.783) (7.5879, -25.8018) (7.559, -25.8207) (7.5301, -25.8397) (7.5014, -25.8588) (7.4728, -25.878) (7.4443, -25.8973) (7.416, -25.9167) (7.3878, -25.9362) (7.3597, -25.9558) (7.3318, -25.9756) (7.304, -25.9954) (7.2763, -26.0153) (7.2488, -26.0354) (7.2214, -26.0555) (7.1941, -26.0758) (7.167, -26.0961) (7.14, -26.1166) (7.1132, -26.1372) (7.0865, -26.1578) (7.0599, -26.1786) (7.0335, -26.1995) (7.0073, -26.2205) (6.9812, -26.2416) (6.9552, -26.2628) (6.9294, -26.2842) (6.9038, -26.3056) (6.8783, -26.3271) (6.8529, -26.3488) (6.8278, -26.3705) (6.8028, -26.3924) (6.7779, -26.4144) (6.7532, -26.4365) (6.7287, -26.4587) (6.7044, -26.481) (6.6802, -26.5034) (6.6562, -26.526) (6.6324, -26.5486) (6.6088, -26.5714) (6.5854, -26.5943) (6.5621, -26.6174) (6.5391, -26.6405) (6.5162, -26.6638) (6.4935, -26.6871) (6.471, -26.7106) (6.4488, -26.7343) (6.4268, -26.7581) (6.405, -26.782) (6.3834, -26.806) (6.362, -26.8302) (6.3409, -26.8545) (6.3199, -26.8789) (6.2992, -26.9034) (6.2787, -26.9281) (6.2585, -26.953) (6.2387, -26.978) (6.2193, -27.0033) (6.2002, -27.0287) (6.1814, -27.0544) (6.1629, -27.0802) (6.1445, -27.106) (6.1264, -27.132) (6.1085, -27.1581) (6.0911, -27.1844) (6.0745, -27.2112) (6.0621, -27.233) (6.0534, -27.2497) (6.0478, -27.261) (6.0451, -27.2667) knots -1 -1 -1 -1 -1 -1 -0.98571429 -0.97142857 -0.95714286 -0.94285714 -0.92857143 -0.91428571 -0.9 -0.88571429 -0.87142857 -0.85714286 -0.84285714 -0.82857143 -0.81428571 -0.8 -0.78571429 -0.77142857 -0.75714286 -0.74285714 -0.72857143 -0.71428571 -0.7 -0.68571429 -0.67142857 -0.65714286 -0.64285714 -0.62857143 -0.61428571 -0.6 -0.58571429 -0.57142857 -0.55714286 -0.54285714 -0.52857143 -0.51428571 -0.5 -0.48571429 -0.47142857 -0.45714286 -0.44285714 -0.42857143 -0.41428571 -0.4 -0.38571429 -0.37142857 -0.35714286 -0.34285714 -0.32857143 -0.31428571 -0.3 -0.28571429 -0.27142857 -0.25714286 -0.24285714 -0.22857143 -0.21428571 -0.2 -0.18571429 -0.17142857 -0.15714286 -0.14285714 -0.12857143 -0.11428571 -0.1 -0.08571429 -0.07142857 -0.05714286 -0.04285714 -0.02857143 -0.01428571 0 0 0 0 0 0
  line L33 (6.0451, -27.2667) -> (5.8737, -27.6268)
  arc A67 (5.5449, -27.747) -> (5.8737, -27.6268) centre (5.648, -27.5193) ccw
  arc A68 (5.5449, -27.747) -> (4.7433, -27.415) centre (0, -40) ccw
  arc A69 (4.5959, -27.0975) -> (4.7433, -27.415) centre (4.8315, -27.1811) ccw
  line L34 (4.5959, -27.0975) -> (4.7292, -26.7217)
  spline S34 degree 5 poles (4.7292, -26.7217) (4.7313, -26.7157) (4.7354, -26.7038) (4.741, -26.6858) (4.7477, -26.6616) (4.7549, -26.6309) (4.7613, -26.6) (4.7671, -26.5689) (4.7726, -26.5377) (4.7779, -26.5065) (4.783, -26.4752) (4.7879, -26.4438) (4.7924, -26.4123) (4.7965, -26.3806) (4.8002, -26.3489) (4.8035, -26.3171) (4.8065, -26.2851) (4.8092, -26.2531) (4.8116, -26.221) (4.8138, -26.1889) (4.8158, -26.1567) (4.8176, -26.1244) (4.8191, -26.0921) (4.8203, -26.0597) (4.8213, -26.0273) (4.822, -25.9948) (4.8225, -25.9622) (4.8228, -25.9296) (4.8228, -25.8969) (4.8227, -25.8642) (4.8223, -25.8314) (4.8217, -25.7986) (4.8209, -25.7658) (4.8199, -25.7328) (4.8187, -25.6999) (4.8172, -25.6669) (4.8156, -25.6339) (4.8138, -25.6008) (4.8118, -25.5677) (4.8095, -25.5345) (4.8071, -25.5014) (4.8045, -25.4681) (4.8017, -25.4349) (4.7987, -25.4016) (4.7956, -25.3683) (4.7922, -25.3349) (4.7887, -25.3016) (4.785, -25.2681) (4.7811, -25.2347) (4.777, -25.2012) (4.7727, -25.1677) (4.7683, -25.1342) (4.7637, -25.1007) (4.7589, -25.0671) (4.754, -25.0335) (4.7488, -24.9999) (4.7435, -24.9662) (4.738, -24.9326) (4.7324, -24.8989) (4.7266, -24.8652) (4.7206, -24.8314) (4.7145, -24.7977) (4.7082, -24.7639) (4.7017, -24.7301) (4.6951, -24.6963) (4.6883, -24.6625) (4.6813, -24.6287) (4.6742, -24.5948) (4.6669, -24.561) (4.6595, -24.5271) (4.6519, -24.4932) (4.6457, -24.4661) (4.6409, -24.4457) (4.6377, -24.4322) (4.6361, -24.4254) knots 0 0 0 0 0 0 0.01428571 0.02857143 0.04285714 0.05714286 0.07142857 0.08571429 0.1 0.11428571 0.12857143 0.14285714 0.15714286 0.17142857 0.18571429 0.2 0.21428571 0.22857143 0.24285714 0.25714286 0.27142857 0.28571429 0.3 0.31428571 0.32857143 0.34285714 0.35714286 0.37142857 0.38571429 0.4 0.41428571 0.42857143 0.44285714 0.45714286 0.47142857 0.48571429 0.5 0.51428571 0.52857143 0.54285714 0.55714286 0.57142857 0.58571429 0.6 0.61428571 0.62857143 0.64285714 0.65714286 0.67142857 0.68571429 0.7 0.71428571 0.72857143 0.74285714 0.75714286 0.77142857 0.78571429 0.8 0.81428571 0.82857143 0.84285714 0.85714286 0.87142857 0.88571429 0.9 0.91428571 0.92857143 0.94285714 0.95714286 0.97142857 0.98571429 1 1 1 1 1 1
  arc A70 (4.6361, -24.4254) -> (3.7723, -24.1939) centre (0, -40) ccw
  spline S35 degree 5 poles (3.7723, -24.1939) (3.7675, -24.199) (3.758, -24.2092) (3.7437, -24.2244) (3.7248, -24.2448) (3.7012, -24.2703) (3.6779, -24.296) (3.6546, -24.3216) (3.6315, -24.3474) (3.6086, -24.3732) (3.5858, -24.3991) (3.5631, -24.4251) (3.5406, -24.4511) (3.5183, -24.4772) (3.4961, -24.5033) (3.4741, -24.5296) (3.4522, -24.5558) (3.4304, -24.5822) (3.4089, -24.6086) (3.3875, -24.6351) (3.3662, -24.6617) (3.3451, -24.6883) (3.3242, -24.715) (3.3034, -24.7417) (3.2828, -24.7685) (3.2624, -24.7954) (3.2421, -24.8223) (3.222, -24.8494) (3.2021, -24.8764) (3.1823, -24.9036) (3.1628, -24.9308) (3.1434, -24.958) (3.1241, -24.9854) (3.1051, -25.0128) (3.0862, -25.0403) (3.0675, -25.0678) (3.0491, -25.0954) (3.0307, -25.123) (3.0126, -25.1508) (2.9947, -25.1786) (2.977, -25.2064) (2.9594, -25.2343) (2.9421, -25.2623) (2.925, -25.2904) (2.9081, -25.3185) (2.8914, -25.3467) (2.8749, -25.375) (2.8586, -25.4033) (2.8425, -25.4317) (2.8266, -25.4601) (2.811, -25.4886) (2.7956, -25.5172) (2.7805, -25.5459) (2.7656, -25.5746) (2.751, -25.6034) (2.7367, -25.6323) (2.7225, -25.6613) (2.7086, -25.6903) (2.6949, -25.7193) (2.6815, -25.7485) (2.6685, -25.7777) (2.6558, -25.807) (2.6435, -25.8365) (2.6317, -25.866) (2.6202, -25.8956) (2.609, -25.9253) (2.5979, -25.9551) (2.5871, -25.9848) (2.5766, -26.0146) (2.5667, -26.0446) (2.5576, -26.0747) (2.5512, -26.0991) (2.5471, -26.1175) (2.5447, -26.1298) (2.5435, -26.136) knots -1 -1 -1 -1 -1 -1 -0.98571429 -0.97142857 -0.95714286 -0.94285714 -0.92857143 -0.91428571 -0.9 -0.88571429 -0.87142857 -0.85714286 -0.84285714 -0.82857143 -0.81428571 -0.8 -0.78571429 -0.77142857 -0.75714286 -0.74285714 -0.72857143 -0.71428571 -0.7 -0.68571429 -0.67142857 -0.65714286 -0.64285714 -0.62857143 -0.61428571 -0.6 -0.58571429 -0.57142857 -0.55714286 -0.54285714 -0.52857143 -0.51428571 -0.5 -0.48571429 -0.47142857 -0.45714286 -0.44285714 -0.42857143 -0.41428571 -0.4 -0.38571429 -0.37142857 -0.35714286 -0.34285714 -0.32857143 -0.31428571 -0.3 -0.28571429 -0.27142857 -0.25714286 -0.24285714 -0.22857143 -0.21428571 -0.2 -0.18571429 -0.17142857 -0.15714286 -0.14285714 -0.12857143 -0.11428571 -0.1 -0.08571429 -0.07142857 -0.05714286 -0.04285714 -0.02857143 -0.01428571 0 0 0 0 0 0
  line L35 (2.5435, -26.136) -> (2.4711, -26.5282)
  arc A71 (2.1846, -26.7294) -> (2.4711, -26.5282) centre (2.2252, -26.4827) ccw
  arc A72 (2.1846, -26.7294) -> (1.3245, -26.6162) centre (0, -40) ccw
  arc A73 (1.0999, -26.3476) -> (1.3245, -26.6162) centre (1.3491, -26.3674) ccw
  line L36 (1.0999, -26.3476) -> (1.1314, -25.9501)
  spline S36 degree 5 poles (1.1314, -25.9501) (1.1319, -25.9438) (1.1327, -25.9313) (1.1335, -25.9124) (1.1337, -25.8873) (1.1327, -25.8558) (1.1308, -25.8243) (1.1284, -25.7928) (1.1257, -25.7612) (1.1227, -25.7297) (1.1196, -25.6981) (1.1161, -25.6665) (1.1123, -25.6349) (1.1081, -25.6033) (1.1035, -25.5717) (1.0984, -25.5401) (1.093, -25.5084) (1.0873, -25.4768) (1.0814, -25.4452) (1.0752, -25.4136) (1.0688, -25.382) (1.0622, -25.3504) (1.0552, -25.3188) (1.048, -25.2872) (1.0406, -25.2556) (1.0329, -25.224) (1.0249, -25.1924) (1.0168, -25.1608) (1.0083, -25.1292) (0.9997, -25.0977) (0.9909, -25.0661) (0.9818, -25.0346) (0.9725, -25.003) (0.963, -24.9715) (0.9533, -24.94) (0.9434, -24.9085) (0.9333, -24.877) (0.923, -24.8455) (0.9124, -24.8141) (0.9017, -24.7826) (0.8908, -24.7512) (0.8797, -24.7198) (0.8684, -24.6884) (0.8569, -24.657) (0.8452, -24.6257) (0.8333, -24.5943) (0.8213, -24.563) (0.809, -24.5317) (0.7966, -24.5004) (0.784, -24.4691) (0.7712, -24.4379) (0.7583, -24.4066) (0.7451, -24.3754) (0.7318, -24.3442) (0.7183, -24.3131) (0.7047, -24.2819) (0.6909, -24.2508) (0.6769, -24.2197) (0.6627, -24.1886) (0.6484, -24.1575) (0.6339, -24.1265) (0.6192, -24.0955) (0.6044, -24.0645) (0.5894, -24.0336) (0.5742, -24.0026) (0.5589, -23.9717) (0.5434, -23.9408) (0.5278, -23.91) (0.512, -23.8792) (0.496, -23.8484) (0.4799, -23.8176) (0.4669, -23.793) (0.4571, -23.7746) (0.4505, -23.7623) (0.4472, -23.7562) knots 0 0 0 0 0 0 0.01428571 0.02857143 0.04285714 0.05714286 0.07142857 0.08571429 0.1 0.11428571 0.12857143 0.14285714 0.15714286 0.17142857 0.18571429 0.2 0.21428571 0.22857143 0.24285714 0.25714286 0.27142857 0.28571429 0.3 0.31428571 0.32857143 0.34285714 0.35714286 0.37142857 0.38571429 0.4 0.41428571 0.42857143 0.44285714 0.45714286 0.47142857 0.48571429 0.5 0.51428571 0.52857143 0.54285714 0.55714286 0.57142857 0.58571429 0.6 0.61428571 0.62857143 0.64285714 0.65714286 0.67142857 0.68571429 0.7 0.71428571 0.72857143 0.74285714 0.75714286 0.77142857 0.78571429 0.8 0.81428571 0.82857143 0.84285714 0.85714286 0.87142857 0.88571429 0.9 0.91428571 0.92857143 0.94285714 0.95714286 0.97142857 0.98571429 1 1 1 1 1 1
  arc A74 (0.4472, -23.7562) -> (-0.4472, -23.7562) centre (0, -40) ccw